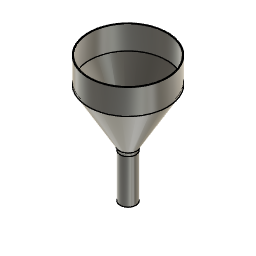
lejek v1 (Autodesk Fusion 360 design; units mm, degrees)
Autodesk Fusion 360 part; units mm, degrees
sketch "Szkic1" plane through (0, 0, 0) normal (0, 0, 1) x (1, 0, 0)
  circle A0 centre (0, 0) radius 9
  circle A1 centre (0, 0) radius 10
  constraint coincident A0.centre A1.centre
extrude "Wyciągnięcie proste1" add sketch "Szkic1" along normal blind 30
extrude "Wyciągnięcie proste2" add 1 faces at (9.6294, -0.4968, 30) along direction (0, 0, 1) blind 60
extrude "Wyciągnięcie proste3" cut 1 faces at (9.6294, -0.4968, 90) along direction (0, 0, -1) blind 30
sketch "Szkic2" plane through (0, 0, 60) normal (0, 0, 1) x (-1, 0, 0)
  circle A0 centre (0, 0) radius 9
  circle A1 centre (0, 0) radius 10
  circle A2 centre (0, 0) radius 50
  dimension "d7" = 100
  constraint concentric A0 A2
  measures "d7" diameter of A2
extrude "Wyciągnięcie proste4" add sketch "Szkic2" along normal blind 100 contours A1 | A2
hole "Otwór1" at (0, 0, 160) direction (0, 0, -1) diameter 98 depth 30 tip angle 60
chamfer "Fazowanie1" distance 68 angle 30 1 edges at (46.6164, 18.0808, 60) measured on face at (-49.7515, 4.9784, 93.3333)
fillet "Zaokrąglenie1" radius 14 1 edges at (-9.3233, 3.6162, 60)
fillet "Zaokrąglenie2" radius 17 1 edges at (-8.3909, -3.2545, 60.718)
